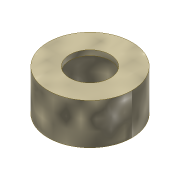
# Autodesk Inventor part: PI_holder
Saved by Autodesk Inventor 2014 (Build 180170000, 170)
## iProperties
Created: 2016-07-07
Part Number: PI_holder
Material: Generic
Document SubType Name: Modeling
Designer: Camilo
Density: 1 g/cm^3
Appearance: Fine - Cream
Author: Camilo
Autodesk Inventor part; units mm, degrees
ref_plane "YZ Plane" through (0, 0, 0) normal (1, 0, 0) x (0, 1, 0)
ref_plane "XZ Plane" through (0, 0, 0) normal (0, 1, 0) x (-1, 0, 0)
ref_plane "XY Plane" through (0, 0, 0) normal (0, 0, 1) x (1, 0, 0)
sketch "Sketch1" plane through (0, 0, 0) normal (0, 0, 1) x (1, 0, 0)
  circle A0 centre (0, 0) radius 8.25 projected
  circle A1 centre (0, 0) radius 9.25
  point P0 (0, 0)
  dimension "d0" = 1
  constraints: 1 centre point
  measures "d0" radial gap between concentric circles of A1 A0
extrude "Extrusion1" add sketch "Sketch1" along normal blind 1.5 contours A0 | A1
sketch "Sketch2" plane through (0, 0, 1.5) normal (0, 0, 1) x (1, 0, 0)
  circle A0 centre (0, 0) radius 9.25 projected
  circle A1 centre (0, 0) radius 12.25
  dimension "d3" = 3
  constraints: 1 centre point
  measures "d3" radial gap between concentric circles of A1 A0
extrude "Extrusion2" add sketch "Sketch2" against normal blind 12
sketch "Sketch3" plane through (0, 0, 1.5) normal (0, 0, 1) x (1, 0, 0)
  circle A0 centre (0, 0) radius 6.94 projected
  circle A1 centre (0, 0) radius 5.94
  dimension "d6" = 1
  constraints: 1 centre point
  measures "d6" radial gap between concentric circles of A0 A1
extrude "Extrusion3" cut sketch "Sketch3" against normal through all contours A1
body "Solid1"
